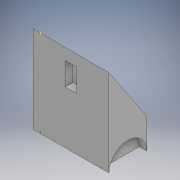
# Autodesk Inventor part: Sumobot v1.0
Saved by Autodesk Inventor 2017 (Build 210142000, 142)
## iProperties
Created: 2021-01-07
Part Number: Sumobot v1.0
Material: Generic
Document SubType Name: Modeling
Designer: ldxcz
Density: 1 g/cm^3
Appearance: Default
Author: ldxcz
Autodesk Inventor part; units mm, degrees
ref_plane "YZ Plane" through (0, 0, 0) normal (1, 0, 0) x (0, 1, 0)
ref_plane "XZ Plane" through (0, 0, 0) normal (0, 1, 0) x (-1, 0, 0)
ref_plane "XY Plane" through (0, 0, 0) normal (0, 0, 1) x (1, 0, 0)
sketch "Sketch1" plane through (0, 0, 0) normal (0, 1, 0) x (-1, 0, 0)
  line L0 (0, 0) -> (200, 0)
  line L1 (200, 0) -> (200, -150)
  line L2 (200, -150) -> (0, -150)
  line L3 (0, -150) -> (0, 0)
  dimension "d0" = 150
  dimension "d1" = 200
  constraints: 8 end point, 2 parallel, 1 horizontal, 1 perpendicular
  measures "d0" distance of L0.end L1.end
  measures "d1" distance of L1.end L2.end
extrude "Extrusion1" add sketch "Sketch1" along normal blind 100
sketch "Sketch4" plane through (0, 0, 0) normal (1, 0, 0) x (0, 0, -1)
  line L0 (0, 100) -> (0, 0)
  line L1 (0, 100) -> (150, 100) projected
  line L2 (0, 0) -> (150, 100)
  line L3 (150, 100) -> (0, 100)
  constraints: 6 end point, 1 collinear, 1 vertical
extrude "Extrusion3" cut sketch "Sketch4" against normal blind 200
sketch "Sketch5" plane through (0, 0, -150) normal (0, 0, -1) x (-1, 0, 0)
  line L0 (0, 0) -> (0, 100) projected
  line L1 (200, 0) -> (0, 0) projected
  line L2 (0, 100) -> (200, 100)
  line L3 (200, 100) -> (200, 0)
  line L4 (200, 0) -> (0, 0)
  line L5 (0, 0) -> (0, 100)
  constraints: 8 end point, 2 parallel, 1 horizontal, 1 perpendicular
extrude "Extrusion4" add sketch "Sketch5" along normal blind 80
sketch "Sketch6" plane through (0, 0, -230) normal (0, 0, -1) x (-1, 0, 0)
  line L0 (25, 80) -> (175, 80)
  line L1 (175, 80) -> (175, 20)
  line L2 (175, 20) -> (25, 20)
  line L3 (25, 20) -> (25, 80)
  line L4 (0, 0) -> (200, 0) projected
  line L5 (200, 100) -> (0, 100) projected
  line L6 (200, 0) -> (200, 100) projected
  line L7 (0, 100) -> (0, 0) projected
  dimension "d11" = 150
  dimension "d12" = 60
  dimension "d13" = 20
  dimension "d14" = 25
  constraints: 8 end point, 2 parallel, 1 horizontal, 1 perpendicular
  measures "d11" distance of L0.start L0.end
  measures "d12" distance of L2.end L0.start
  measures "d13" distance between parallel lines of L0 L5
  measures "d14" distance between parallel lines of L6 L1
extrude "Extrusion5" cut sketch "Sketch6" against normal blind 75 contours L0 L1 L2 L3
sketch "Sketch7" plane through (0, 0, -155) normal (0, 0, -1) x (-1, 0, 0)
  line L0 (25, 20) -> (25, 80) projected
  line L1 (175, 80) -> (175, 20) projected
  line L2 (25, 20) -> (25, 80) projected
  line L3 (25, 80) -> (175, 80) projected
  line L4 (175, 80) -> (175, 20) projected
  line L5 (175, 20) -> (25, 20) projected
  line L6 (200, 0) -> (200, 100) projected
  line L7 (200, 100) -> (0, 100) projected
  line L8 (0, 100) -> (0, 0) projected
  line L9 (0, 0) -> (200, 0) projected
  line L10 (175, 20) -> (25, 20) projected
  line L11 (25, 80) -> (175, 80) projected
  line L12 (25, 20) -> (25, 80) projected
  line L13 (175, 20) -> (25, 20) projected
  line L14 (175, 80) -> (175, 20) projected
  line L15 (75, 50) -> (125, 50)
  line L16 (125, 50) -> (125, 20)
  line L17 (125, 20) -> (75, 20)
  line L18 (75, 20) -> (75, 50)
  point P0 (0, 0)
  dimension "d17" = 50
  dimension "d18" = 30
  dimension "d20" = 0
  dimension "d21" = 50
  constraints: 8 end point, 2 parallel, 1 horizontal, 1 perpendicular
  measures "d17" distance of L15.start L15.end
  measures "d18" distance of L15.end L16.end
  measures "d20" distance between parallel lines of L5 L17
  measures "d21" distance between parallel lines of L1 L16
extrude "Extrusion6" cut sketch "Sketch7" against normal up to next contours L18 L15 L16 L5
sketch "Sketch8" plane through (-175, 20, -230) normal (0, 1, 0) x (1, 0, 0)
  line L0 (100, -200) -> (50, -200) projected
  line L1 (100, -155) -> (100, -200) projected
  line L2 (50, -200) -> (50, -155) projected
  line L3 (50, -155) -> (100, -155) projected
  line L4 (100, -155) -> (100, -200) projected
  line L5 (100, -200) -> (50, -200) projected
  line L6 (50, -200) -> (50, -155) projected
  line L7 (50, -155) -> (100, -155) projected
  line L8 (175, -80) -> (175, -230) projected
  line L9 (175, -80) -> (-25, -80) projected
  line L10 (-25, -230) -> (-25, -80) projected
  line L11 (175, -230) -> (-25, -230) projected
  line L12 (90, -200) -> (60, -200)
  line L13 (60, -200) -> (60, -140)
  line L14 (60, -140) -> (90, -140)
  line L15 (90, -140) -> (90, -200)
  dimension "d24" = 30
  dimension "d25" = 60
  dimension "d26" = 0
  dimension "d27" = 10
  constraints: 8 end point, 2 parallel, 1 horizontal, 1 perpendicular
  measures "d24" distance of L12.start L12.end
  measures "d25" distance of L12.end L13.end
  measures "d26" distance between parallel lines of L0 L12
  measures "d27" distance between parallel lines of L1 L15
extrude "Extrusion7" cut sketch "Sketch8" against normal up to next contours L0 L13 L3 L15 | L3 L13 L14 L15
sketch "Sketch9" plane through (0, 0, -230) normal (1, 0, 0) x (0, 0, -1)
  line L0 (0, 100) -> (0, 0) projected
  circle A0 centre (0, 50) radius 50
  point P0 (-230, 0)
  dimension "d30" = 100
  constraints: 1 midpoint, 1 vertical alignment, 2 other
extrude "Extrusion8" cut sketch "Sketch9" against normal blind 20
sketch "Sketch10" plane through (-200, 0, -230) normal (-1, 0, 0) x (0, 0, 1)
  circle A0 centre (0, 50) radius 50
  line L0 (0, 0) -> (0, 100) projected
  line L1 (230, 0) -> (0, 0) projected
  dimension "d33" = 100
  constraints: 1 centre point, 1 midpoint, 1 tangent
  measures "d33" diameter of A0
extrude "Extrusion9" cut sketch "Sketch10" against normal blind 20
sketch "Sketch12" plane through (-180, 0, -230) normal (-1, 0, 0) x (0, 0, 1)
  point P0 (230, 0)
body "Solid1"
